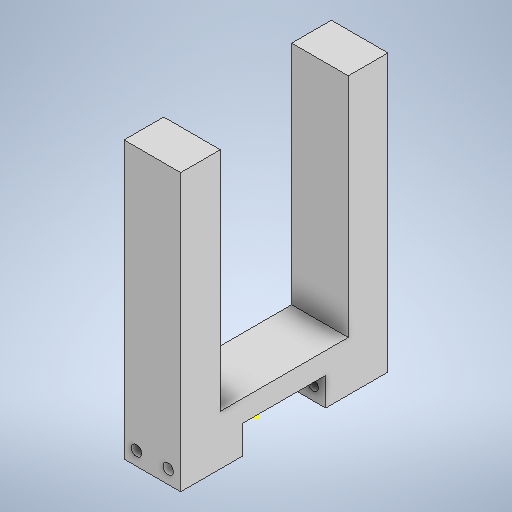
# Autodesk Inventor part: 13042026-10
Saved by Autodesk Inventor 2025.2 (Build 292293000, 293)
## iProperties
Created: 2026-05-05
Part Number: 13042026-10
Material: Generic
Document SubType Name: Modeling
Designer: Oski
Density: 1 g/cm^3
Appearance: Default
Author: Oski
Autodesk Inventor part; units mm, degrees
ref_plane "YZ Plane" through (0, 0, 0) normal (1, 0, 0) x (0, 1, 0)
ref_plane "XZ Plane" through (0, 0, 0) normal (0, 1, 0) x (-1, 0, 0)
ref_plane "XY Plane" through (0, 0, 0) normal (0, 0, 1) x (1, 0, 0)
sketch "Sketch2" plane through (0, 0, 0) normal (0, 0, 1) x (1, 0, 0)
  line L0 (-25, 12) -> (25, 12)
  line L1 (25, 12) -> (25, -12)
  line L2 (25, -12) -> (-25, -12)
  line L3 (-25, -12) -> (-25, 12)
  line L4 (-25, 12) -> (25, -12) construction
  line L5 (25, 12) -> (-25, -12) construction
  point P0 (0, 0)
  dimension "d4" = 24
  dimension "d5" = 50
  constraints: 12 end point, 2 midpoint, 2 parallel, 1 horizontal, 1 perpendicular
  measures "d4" distance of L0.end L1.end
  measures "d5" distance of L1.end L2.end
extrude "Extrusion1" add sketch "Sketch2" along normal mid plane 183
sketch "Sketch5" plane through (0, 0, -91.5) normal (0, 0, -1) x (-1, 0, 0)
  line L0 (-14, 0) -> (-25, 0) construction
  line L1 (-25, -12) -> (-25, 12) projected
  line L2 (14, 0) -> (25, 0) construction
  line L3 (25, 12) -> (25, -12) projected
  line L4 (-25, 0) -> (25, 0) construction
  point P0 (0, 0)
  dimension "d14" = 28
  constraints: 6 end point, 2 midpoint, 2 point on line, 1 collinear, 1 horizontal
  measures "d14" distance of L0.start L2.start
hole "Hole1" at (-14, 0, -91.5) direction (0, 0, 1) diameter 9.2 end through all
hole "Hole2" at (14, 0, -91.5) direction (0, 0, 1) diameter 9.2 end through all
sketch "Sketch6" plane through (-25, -12, -91.5) normal (0, -1, 0) x (1, 0, 0)
  point P0 (25, 91.5)
sketch "Sketch7" plane through (-25, -12, 91.5) normal (0, -1, 0) x (1, 0, 0)
  line L0 (50, -55) -> (0, -55)
  line L1 (0, -55) -> (0, -128)
  line L2 (0, -128) -> (50, -128)
  line L3 (50, -128) -> (50, -55)
  line L4 (50, -55) -> (0, -128) construction
  line L5 (0, -55) -> (50, -128) construction
  line L6 (25, -128) -> (25, -183) construction
  line L7 (50, -183) -> (0, -183) projected
  line L8 (25, -55) -> (25, 0) construction
  line L9 (0, 0) -> (0, -183) projected
  point P0 (25, -91.5)
  dimension "d30" = 55
  constraints: 16 end point, 5 midpoint, 2 parallel, 2 point on line, 1 collinear, 1 horizontal, 1 perpendicular
  measures "d30" distance of L6.start L6.end
sketch "Sketch8" plane through (-25, 12, 91.5) normal (0, 1, 0) x (1, 0, 0)
  line L0 (50, 183) -> (50, 0) projected
  line L1 (0, 35) -> (50, 35)
  line L2 (50, 35) -> (50, 148)
  line L3 (50, 148) -> (0, 148)
  line L4 (0, 148) -> (0, 35)
  line L5 (0, 35) -> (50, 148) construction
  line L6 (50, 35) -> (0, 148) construction
  line L7 (0, 183) -> (50, 183) projected
  point P0 (25, 91.5)
  dimension "d31" = 35
  constraints: 12 end point, 2 midpoint, 2 parallel, 1 horizontal, 1 perpendicular, 1 point on line
  measures "d31" distance between parallel lines of L7 L3
extrude "Extrusion4" add sketch "Sketch8" along normal blind 20
extrude "Extrusion5" cut sketch "Sketch7" against normal blind 25
sketch "Sketch9" plane through (-25, 12, 91.5) normal (0, 1, 0) x (1, 0, 0)
  line L0 (0, 35) -> (50, 35) projected
  line L1 (50, 35) -> (0, 35)
  line L2 (0, 35) -> (0, 0)
  line L3 (0, 0) -> (50, 0)
  line L4 (50, 0) -> (50, 35)
  point P0 (25, 91.5)
  constraints: 8 end point, 2 parallel, 1 horizontal, 1 perpendicular
extrude "Extrusion6" add sketch "Sketch9" along normal blind 220
sketch "Sketch10" plane through (-25, 12, -91.5) normal (0, 1, 0) x (1, 0, 0)
  line L0 (50, 0) -> (50, -35) projected
  line L1 (50, 0) -> (0, 0)
  line L2 (0, 0) -> (0, -35)
  line L3 (0, -35) -> (50, -35)
  line L4 (50, -35) -> (50, 0)
  point P0 (25, -91.5)
  constraints: 8 end point, 2 parallel, 1 horizontal, 1 perpendicular
extrude "Extrusion7" add sketch "Sketch10" along normal blind 220
body "Solid1"
